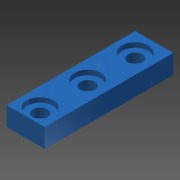
# Autodesk Inventor part: XCarriageBeltClampRight
Saved by Autodesk Inventor 2015 (Build 190159000, 159)
## iProperties
Created: 2014-08-22
Part Number: XCarriageBeltClampRight
Material: ABS Plastic
Document SubType Name: Modeling
Designer: t_clevj
Density: 1.06 g/cm^3
Appearance: Cyan
Author: t_clevj
Autodesk Inventor part; units mm, degrees
ref_plane "YZ Plane" through (0, 0, 0) normal (1, 0, 0) x (0, 1, 0)
ref_plane "XZ Plane" through (0, 0, 0) normal (0, 1, 0) x (-1, 0, 0)
ref_plane "XY Plane" through (0, 0, 0) normal (0, 0, 1) x (1, 0, 0)
sketch "Sketch1" plane through (0, 0, 0) normal (0, 0, 1) x (1, 0, 0)
  line L0 (0, 0) -> (8, 0)
  line L1 (8, 0) -> (8, 27)
  line L2 (8, 27) -> (0, 27)
  line L3 (0, 27) -> (0, 0)
  dimension "d0" = 27
  dimension "d1" = 8
  constraints: 8 end point, 2 parallel, 1 horizontal, 1 perpendicular
  measures "d0" distance of L2.end L0.start
  measures "d1" distance of L0.start L0.end
extrude "Extrusion1" add sketch "Sketch1" along normal blind 4
sketch "Sketch2" plane through (0, 0, 4) normal (0, 0, 1) x (1, 0, 0)
  line L0 (0, 0) -> (8, 0) projected
  line L1 (8, 0) -> (8, 27) projected
  point P0 (4, 23)
  point P1 (4, 13)
  point P2 (4, 3)
  dimension "d4" = 3
  dimension "d5" = 20
  dimension "d6" = 10
  dimension "d7" = 4
  constraints: 2 vertical alignment
  measures "d4" distance from line of L0 point (4, 3)
  measures "d5" distance of point (4, 23) point (4, 3)
  measures "d6" distance of point (4, 3) point (4, 13)
  measures "d7" distance from line of L1 point (4, 3)
hole "Hole1" at (4, 23, 4) at (4, 13, 4) at (4, 3, 4) direction (0, 0, -1) diameter 3 end up to face face through (2.6667, 18, 0) facing (0, 0, -1) counterbore diameter 5.5 counterbore depth 1
body "Solid1"
